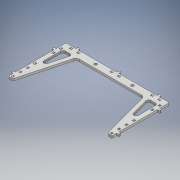
# Autodesk Inventor part: turtlebot_installation_fin_top
Saved by Autodesk Inventor 2018 (Build 220112000, 112)
## iProperties
Created: 2018-07-16
Part Number: turtlebot_installation_fin_top
Material: Generic
Document SubType Name: Modeling
Designer: Tsche
Density: 1 g/cm^3
Appearance: Default
Author: Tsche
Autodesk Inventor part; units mm, degrees
ref_plane "YZ Plane" through (0, 0, 0) normal (1, 0, 0) x (0, 1, 0)
ref_plane "XZ Plane" through (0, 0, 0) normal (0, 1, 0) x (-1, 0, 0)
ref_plane "XY Plane" through (0, 0, 0) normal (0, 0, 1) x (1, 0, 0)
sketch "Sketch1" plane through (0, 0, 0) normal (0, 0, 1) x (1, 0, 0)
  line L0 (0, 0) -> (1.5, 0) construction
  line L1 (70, 0) -> (70, -13.5)
  line L2 (70, -78) -> (64, -78)
  line L3 (64, -78) -> (45.7795, -10)
  line L4 (45.7795, -10) -> (0, -10)
  line L5 (-102.2, 0) -> (102.2, 0) construction
  line L6 (0, -94.2) -> (0, 19.2) construction
  line L7 (70, -71.5) -> (73, -71.5)
  line L8 (73, -71.5) -> (73, -68.5)
  line L9 (73, -68.5) -> (70, -68.5)
  line L10 (70, -13.5) -> (73, -13.5)
  line L11 (73, -13.5) -> (73, -16.5)
  line L12 (73, -16.5) -> (70, -16.5)
  line L13 (70, -13.5) -> (70, -16.5) construction
  line L14 (70, -16.5) -> (70, -68.5)
  line L15 (70, -68.5) -> (70, -71.5) construction
  line L16 (70, -71.5) -> (70, -78)
  line L17 (70, -70) -> (73, -70) construction
  line L18 (70, -15) -> (73, -15) construction
  line L19 (65.7, -73.5) -> (67, -73.5)
  line L20 (67, -73.5) -> (67, -76.5)
  line L21 (67, -76.5) -> (65.7, -76.5)
  line L22 (65.7, -76.5) -> (65.7, -73.5)
  line L23 (65.7, -75) -> (67, -75) construction
  line L24 (65.7, -66.5) -> (67, -66.5)
  line L25 (67, -66.5) -> (67, -63.5)
  line L26 (67, -63.5) -> (65.7, -63.5)
  line L27 (65.7, -63.5) -> (65.7, -66.5)
  line L28 (65.7, -65) -> (67, -65) construction
  line L29 (67, -8.5) -> (65.7, -8.5)
  line L30 (65.7, -10) -> (67, -10) construction
  line L31 (67, -11.5) -> (67, -8.5)
  line L32 (65.7, -11.5) -> (67, -11.5)
  line L33 (65.7, -8.5) -> (65.7, -11.5)
  line L34 (65.7, -18.5) -> (67, -18.5)
  line L35 (65.7, -20) -> (67, -20) construction
  line L36 (67, -18.5) -> (67, -21.5)
  line L37 (67, -21.5) -> (65.7, -21.5)
  line L38 (65.7, -21.5) -> (65.7, -18.5)
  line L39 (65.7, -53.5) -> (67, -53.5)
  line L40 (67, -53.5) -> (67, -56.5)
  line L41 (67, -56.5) -> (65.7, -56.5)
  line L42 (65.7, -56.5) -> (65.7, -53.5)
  line L43 (70, -50) -> (67.2, -50) construction
  line L44 (65.7, -55) -> (67, -55) construction
  line L45 (65.7, -46.5) -> (67, -46.5)
  line L46 (67, -46.5) -> (67, -43.5)
  line L47 (67, -43.5) -> (65.7, -43.5)
  line L48 (65.7, -43.5) -> (65.7, -46.5)
  line L49 (65.7, -45) -> (67, -45) construction
  line L50 (0, 3) -> (1.5, 3)
  line L51 (1.5, 3) -> (1.5, 0)
  line L52 (1.5, 0) -> (53.5, 0)
  line L53 (56.5, 0) -> (56.5, 3)
  line L54 (56.5, 3) -> (53.5, 3)
  line L55 (53.5, 3) -> (53.5, 0)
  line L56 (53.5, 0) -> (56.5, 0) construction
  line L57 (56.5, 0) -> (70, 0)
  line L58 (55, 3) -> (55, 0) construction
  line L59 (3.5, -3) -> (6.5, -3)
  line L60 (6.5, -3) -> (6.5, -4.3)
  line L61 (6.5, -4.3) -> (3.5, -4.3)
  line L62 (3.5, -4.3) -> (3.5, -3)
  line L63 (5, -3) -> (5, -4.3) construction
  line L64 (51.5, -3) -> (51.5, -4.3)
  line L65 (50, -3) -> (50, -4.3) construction
  line L66 (51.5, -4.3) -> (48.5, -4.3)
  line L67 (48.5, -3) -> (51.5, -3)
  line L68 (48.5, -4.3) -> (48.5, -3)
  line L69 (58.5, -3) -> (58.5, -4.3)
  line L70 (60, -3) -> (60, -4.3) construction
  line L71 (58.5, -4.3) -> (61.5, -4.3)
  line L72 (61.5, -3) -> (58.5, -3)
  line L73 (61.5, -4.3) -> (61.5, -3)
  line L74 (0, 0) -> (-1.5, 0) construction
  line L75 (-70, 0) -> (-70, -13.5)
  line L76 (-70, -78) -> (-64, -78)
  line L77 (-64, -78) -> (-45.7795, -10)
  line L78 (-45.7795, -10) -> (0, -10)
  line L79 (-70, -71.5) -> (-73, -71.5)
  line L80 (-73, -71.5) -> (-73, -68.5)
  line L81 (-73, -68.5) -> (-70, -68.5)
  line L82 (-70, -13.5) -> (-73, -13.5)
  line L83 (-73, -13.5) -> (-73, -16.5)
  line L84 (-73, -16.5) -> (-70, -16.5)
  line L85 (-70, -13.5) -> (-70, -16.5) construction
  line L86 (-70, -16.5) -> (-70, -68.5)
  line L87 (-70, -68.5) -> (-70, -71.5) construction
  line L88 (-70, -71.5) -> (-70, -78)
  line L89 (-70, -70) -> (-73, -70) construction
  line L90 (-70, -15) -> (-73, -15) construction
  line L91 (-65.7, -73.5) -> (-67, -73.5)
  line L92 (-67, -73.5) -> (-67, -76.5)
  line L93 (-67, -76.5) -> (-65.7, -76.5)
  line L94 (-65.7, -76.5) -> (-65.7, -73.5)
  line L95 (-65.7, -75) -> (-67, -75) construction
  line L96 (-65.7, -66.5) -> (-67, -66.5)
  line L97 (-65.7, -65) -> (-67, -65) construction
  line L98 (-67, -66.5) -> (-67, -63.5)
  line L99 (-67, -63.5) -> (-65.7, -63.5)
  line L100 (-65.7, -63.5) -> (-65.7, -66.5)
  line L101 (-67, -8.5) -> (-65.7, -8.5)
  line L102 (-65.7, -10) -> (-67, -10) construction
  line L103 (-67, -11.5) -> (-67, -8.5)
  line L104 (-65.7, -11.5) -> (-67, -11.5)
  line L105 (-65.7, -8.5) -> (-65.7, -11.5)
  line L106 (-65.7, -18.5) -> (-67, -18.5)
  line L107 (-65.7, -20) -> (-67, -20) construction
  line L108 (-67, -18.5) -> (-67, -21.5)
  line L109 (-67, -21.5) -> (-65.7, -21.5)
  line L110 (-65.7, -21.5) -> (-65.7, -18.5)
  line L111 (-65.7, -53.5) -> (-67, -53.5)
  line L112 (-67, -53.5) -> (-67, -56.5)
  line L113 (-67, -56.5) -> (-65.7, -56.5)
  line L114 (-65.7, -56.5) -> (-65.7, -53.5)
  line L115 (-70, -50) -> (-67.2, -50) construction
  line L116 (-65.7, -55) -> (-67, -55) construction
  line L117 (-67, -43.5) -> (-65.7, -43.5)
  line L118 (-65.7, -45) -> (-67, -45) construction
  line L119 (-67, -46.5) -> (-67, -43.5)
  line L120 (-65.7, -43.5) -> (-65.7, -46.5)
  line L121 (-65.7, -46.5) -> (-67, -46.5)
  line L122 (0, 3) -> (-1.5, 3)
  line L123 (-1.5, 3) -> (-1.5, 0)
  line L124 (-1.5, 0) -> (-53.5, 0)
  line L125 (-56.5, 0) -> (-56.5, 3)
  line L126 (-56.5, 3) -> (-53.5, 3)
  line L127 (-53.5, 3) -> (-53.5, 0)
  line L128 (-53.5, 0) -> (-56.5, 0) construction
  line L129 (-56.5, 0) -> (-70, 0)
  line L130 (-55, 3) -> (-55, 0) construction
  line L131 (-3.5, -3) -> (-6.5, -3)
  line L132 (-6.5, -3) -> (-6.5, -4.3)
  line L133 (-6.5, -4.3) -> (-3.5, -4.3)
  line L134 (-3.5, -4.3) -> (-3.5, -3)
  line L135 (-5, -3) -> (-5, -4.3) construction
  line L136 (-51.5, -3) -> (-51.5, -4.3)
  line L137 (-50, -3) -> (-50, -4.3) construction
  line L138 (-51.5, -4.3) -> (-48.5, -4.3)
  line L139 (-48.5, -3) -> (-51.5, -3)
  line L140 (-48.5, -4.3) -> (-48.5, -3)
  line L141 (-58.5, -3) -> (-58.5, -4.3)
  line L142 (-60, -3) -> (-60, -4.3) construction
  line L143 (-58.5, -4.3) -> (-61.5, -4.3)
  line L144 (-61.5, -3) -> (-58.5, -3)
  line L145 (-61.5, -4.3) -> (-61.5, -3)
  line L146 (50.9558, -10) -> (64, -10)
  line L147 (64, -10) -> (64, -58.6815)
  line L148 (64, -58.6815) -> (50.9558, -10)
  line L149 (-50.9558, -10) -> (-64, -10)
  line L150 (-64, -10) -> (-64, -58.6815)
  line L151 (-64, -58.6815) -> (-50.9558, -10)
  circle A0 centre (-25, -5) radius 1.85
  circle A1 centre (25, -5) radius 1.85
  dimension "d1" = 10
  dimension "d2" = 6
  dimension "d3" = 15
  dimension "d5" = 70
  dimension "d6" = 3
  dimension "d8" = 8
  dimension "d9" = 15
  dimension "d10" = 55
  dimension "d11" = 5
  dimension "d12" = 3
  dimension "d13" = 1.3
  dimension "d14" = 3
  dimension "d17" = 55
  dimension "d25" = 5
  dimension "d26" = 3
  dimension "d27" = 1.3
  dimension "d28" = 3
  dimension "d29" = 50
  dimension "d30" = 1.5
  dimension "d31" = 15
  dimension "d32" = 5
  dimension "d33" = 3
  dimension "d34" = 5
  dimension "d37" = 45
  dimension "d42" = 5
  dimension "d47" = 6
  dimension "d48" = 5
  dimension "d51" = 5
  dimension "d52" = 3.7
  dimension "d53" = 25
  constraints: 300 end point, 102 symmetric about line, 45 perpendicular, 18 point on line, 13 horizontal, 12 midpoint, 11 parallel, 6 equal length, 3 collinear, 2 centre point, 1 vertical, 34 other
  measures "d1" distance between parallel lines of L0 L4
  measures "d2" distance of L2.start L2.end
  measures "d3" angle of L1 L3
  measures "d5" distance between parallel lines of L14 L6
  measures "d6" distance of L10.end L11.end
  measures "d8" distance between parallel lines of L2 L17
  measures "d9" distance between parallel lines of L0 L18
  measures "d10" distance between parallel lines of L18 L17
  measures "d11" distance between parallel lines of L17 L23
  measures "d12" distance between parallel lines of L16 L20
  measures "d13" distance of L19.start L19.end
  measures "d14" distance of L21.end L19.start
  measures "d17" distance of L25.end L29.start
  measures "d25" distance between parallel lines of L43 L44
  measures "d26" distance of L41.end L39.start
  measures "d27" distance of L40.end L41.end
  measures "d28" distance between parallel lines of L14 L40
  measures "d29" distance between parallel lines of L5 L43
  measures "d30" distance between parallel lines of L6 L51
  measures "d31" distance between parallel lines of L58 L1
  measures "d32" distance between parallel lines of L18 L30
  measures "d33" distance between parallel lines of L5 L59
  measures "d34" distance between parallel lines of L6 L63
  measures "d37" distance of L60.end L64.end
  measures "d42" distance between parallel lines of L58 L65
  measures "d47" distance between parallel lines of L14 L147
  measures "d48" distance between parallel lines of L3 L148
  measures "d51" distance from line of A0.centre L5
  measures "d52" diameter of A0
  measures "d53" distance from line of L6 A0.centre
extrude "Extrusion1" add sketch "Sketch1" along normal blind 3
fillet "Fillet1" radius 1 18 edges at (53.5, 3, 1.5) (56.5, 3, 1.5) (1.5, 3, 1.5) (-1.5, 3, 1.5) (-53.5, 3, 1.5) (-56.5, 3, 1.5) (73, -13.5, 1.5) (73, -16.5, 1.5) (73, -68.5, 1.5) (73, -71.5, 1.5) (70, -78, 1.5) (-70, -78, 1.5) (-73, -71.5, 1.5) (-73, -68.5, 1.5) (-73, -16.5, 1.5) (-73, -13.5, 1.5) (-70, 0, 1.5) (70, 0, 1.5)
chamfer "Chamfer1" distance 1 angle 45 36 edges at (-60, -3, 3) (-50, -3, 3) (-60, -3, 0) (-50, -3, 0) (-67, -10, 3) (-67, -10, 0) (-67, -20, 3) (-67, -20, 0) (-67, -55, 3) (-67, -55, 0) (-67, -45, 3) (-67, -45, 0) (-67, -65, 3) (-67, -65, 0) (-67, -75, 3) (-67, -75, 0) (67, -75, 3) (67, -75, 0) (67, -65, 3) (67, -65, 0) (67, -55, 3) (67, -55, 0) (67, -45, 3) (67, -45, 0) (67, -20, 3) (67, -20, 0) (67, -10, 3) (67, -10, 0) (50, -3, 3) (50, -3, 0) (60, -3, 3) (60, -3, 0) (5, -3, 3) (5, -3, 0) (-5, -3, 3) (-5, -3, 0)
fillet "Fillet2" radius 3 8 edges at (-64, -58.6815, 1.5) (-64, -10, 1.5) (-50.9558, -10, 1.5) (50.9558, -10, 1.5) (64, -10, 1.5) (64, -58.6815, 1.5) (-64, -78, 1.5) (64, -78, 1.5)
fillet "Fillet3" radius 5 2 edges at (-45.7795, -10, 1.5) (45.7795, -10, 1.5)
body "Solid1"
